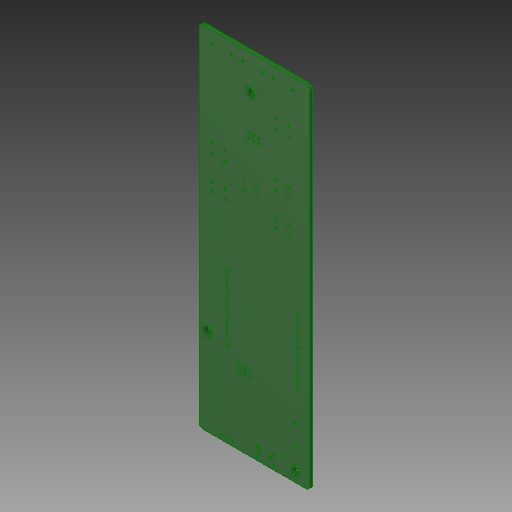
# Autodesk Inventor part: fantimote.kicad_pcb_Kontur
Saved by Autodesk Inventor 2019 (Build 230136000, 136)
## iProperties
Created: 2018-07-30
Part Number: fantimote.kicad_pcb_Kontur
Material: Generisch
Document SubType Name: Modeling
Designer: marc
Density: 1 g/cm^3
Appearance: Board-Kontur
Author: marc
Autodesk Inventor part; units mm, degrees
ref_plane "YZ Plane" through (0, 0, 0) normal (1, 0, 0) x (0, 1, 0)
ref_plane "XZ Plane" through (0, 0, 0) normal (0, 1, 0) x (-1, 0, 0)
ref_plane "XY Plane" through (0, 0, 0) normal (0, 0, 1) x (1, 0, 0)
sketch "Skizze1" plane through (0, 0, 0) normal (0, 0, 1) x (1, 0, 0)
  arc A0 (40.64, -188.595) -> (42.545, -190.5) centre (42.545, -188.595) ccw
  line L0 (42.545, -190.5) -> (93.98, -190.5)
  arc A1 (93.98, -190.5) -> (95.885, -188.595) centre (93.98, -188.595) ccw
  line L1 (95.885, -188.595) -> (95.885, -17.78)
  arc A2 (95.885, -17.78) -> (93.98, -15.875) centre (93.98, -17.78) ccw
  line L2 (93.98, -15.875) -> (42.545, -15.875)
  arc A3 (42.545, -15.875) -> (40.64, -17.78) centre (42.545, -17.78) ccw
  line L3 (40.64, -17.78) -> (40.64, -188.595)
  line L4 (70.36, -184.565) -> (70.36, -185.115)
  arc A4 (69.51, -185.115) -> (70.36, -185.115) centre (69.935, -185.115) ccw
  line L5 (69.51, -185.115) -> (69.51, -184.565)
  arc A5 (70.36, -184.565) -> (69.51, -184.565) centre (69.935, -184.565) ccw
  line L6 (77.81, -184.565) -> (77.81, -185.115)
  arc A6 (76.96, -185.115) -> (77.81, -185.115) centre (77.385, -185.115) ccw
  line L7 (76.96, -185.115) -> (76.96, -184.565)
  arc A7 (77.81, -184.565) -> (76.96, -184.565) centre (77.385, -184.565) ccw
  line L8 (70.06, -188.315) -> (70.06, -188.965)
  arc A8 (69.51, -188.965) -> (70.06, -188.965) centre (69.785, -188.965) ccw
  line L9 (69.51, -188.965) -> (69.51, -188.315)
  arc A9 (70.06, -188.315) -> (69.51, -188.315) centre (69.785, -188.315) ccw
  line L10 (77.81, -188.315) -> (77.81, -188.965)
  arc A10 (77.26, -188.965) -> (77.81, -188.965) centre (77.535, -188.965) ccw
  line L11 (77.26, -188.965) -> (77.26, -188.315)
  arc A11 (77.81, -188.315) -> (77.26, -188.315) centre (77.535, -188.315) ccw
  circle A12 centre (53.49, -85.78) radius 0.5
  circle A13 centre (46.99, -85.78) radius 0.5
  circle A14 centre (53.49, -81.28) radius 0.5
  circle A15 centre (46.99, -81.28) radius 0.5
  circle A16 centre (53.49, -69.27) radius 0.5
  circle A17 centre (46.99, -69.27) radius 0.5
  circle A18 centre (53.49, -64.77) radius 0.5
  circle A19 centre (46.99, -64.77) radius 0.5
  circle A20 centre (47.07, -21.59) radius 0.6
  circle A21 centre (57.07, -21.59) radius 0.6
  circle A22 centre (62.31, -21.59) radius 0.6
  circle A23 centre (72.31, -21.59) radius 0.6
  circle A24 centre (77.55, -21.59) radius 0.6
  circle A25 centre (87.55, -21.59) radius 0.6
  circle A26 centre (70.485, -53.34) radius 0.5
  circle A27 centre (70.485, -50.8) radius 0.5
  circle A28 centre (67.945, -53.34) radius 0.5
  circle A29 centre (67.945, -50.8) radius 0.5
  circle A30 centre (65.405, -53.34) radius 0.5
  circle A31 centre (65.405, -50.8) radius 0.5
  circle A32 centre (54.61, -115.57) radius 0.5
  circle A33 centre (54.61, -118.11) radius 0.5
  circle A34 centre (54.61, -120.65) radius 0.5
  circle A35 centre (54.61, -123.19) radius 0.5
  circle A36 centre (54.61, -125.73) radius 0.5
  circle A37 centre (54.61, -128.27) radius 0.5
  circle A38 centre (54.61, -130.81) radius 0.5
  circle A39 centre (54.61, -133.35) radius 0.5
  circle A40 centre (54.61, -135.89) radius 0.5
  circle A41 centre (54.61, -138.43) radius 0.5
  circle A42 centre (54.61, -140.97) radius 0.5
  circle A43 centre (54.61, -143.51) radius 0.5
  circle A44 centre (54.61, -146.05) radius 0.5
  circle A45 centre (54.61, -148.59) radius 0.5
  circle A46 centre (90.17, -116.205) radius 0.5
  circle A47 centre (90.17, -118.745) radius 0.5
  circle A48 centre (90.17, -121.285) radius 0.5
  circle A49 centre (90.17, -123.825) radius 0.5
  circle A50 centre (90.17, -126.365) radius 0.5
  circle A51 centre (90.17, -128.905) radius 0.5
  circle A52 centre (90.17, -131.445) radius 0.5
  circle A53 centre (90.17, -133.985) radius 0.5
  circle A54 centre (90.17, -136.525) radius 0.5
  circle A55 centre (90.17, -139.065) radius 0.5
  circle A56 centre (90.17, -141.605) radius 0.5
  circle A57 centre (90.17, -144.145) radius 0.5
  circle A58 centre (90.17, -146.685) radius 0.5
  circle A59 centre (90.17, -149.225) radius 0.5
  circle A60 centre (60.96, -153.67) radius 0.5
  circle A61 centre (60.96, -156.21) radius 0.5
  circle A62 centre (63.5, -153.67) radius 0.5
  circle A63 centre (63.5, -156.21) radius 0.5
  circle A64 centre (66.04, -153.67) radius 0.5
  circle A65 centre (66.04, -156.21) radius 0.5
  circle A66 centre (88.9, -175.1813) radius 0.5005
  circle A67 centre (88.9, -165.1787) radius 0.5005
  circle A68 centre (62.715, -72.335) radius 0.5
  circle A69 centre (69.215, -72.335) radius 0.5
  circle A70 centre (62.715, -76.835) radius 0.5
  circle A71 centre (69.215, -76.835) radius 0.5
  circle A72 centre (85.24, -42.6) radius 0.5
  circle A73 centre (78.74, -42.6) radius 0.5
  circle A74 centre (85.24, -38.1) radius 0.5
  circle A75 centre (78.74, -38.1) radius 0.5
  circle A76 centre (45.085, -146.685) radius 1.6
  circle A77 centre (47.485, -146.685) radius 0.25
  circle A78 centre (46.7821, -148.3821) radius 0.25
  circle A79 centre (45.085, -149.085) radius 0.25
  circle A80 centre (43.3879, -148.3821) radius 0.25
  circle A81 centre (42.685, -146.685) radius 0.25
  circle A82 centre (43.3879, -144.9879) radius 0.25
  circle A83 centre (45.085, -144.285) radius 0.25
  circle A84 centre (46.7821, -144.9879) radius 0.25
  circle A85 centre (88.9, -185.42) radius 1.6
  circle A86 centre (91.3, -185.42) radius 0.25
  circle A87 centre (90.5971, -187.1171) radius 0.25
  circle A88 centre (88.9, -187.82) radius 0.25
  circle A89 centre (87.2029, -187.1171) radius 0.25
  circle A90 centre (86.5, -185.42) radius 0.25
  circle A91 centre (87.2029, -183.7229) radius 0.25
  circle A92 centre (88.9, -183.02) radius 0.25
  circle A93 centre (90.5971, -183.7229) radius 0.25
  circle A94 centre (66.675, -33.02) radius 1.6
  circle A95 centre (69.075, -33.02) radius 0.25
  circle A96 centre (68.3721, -34.7171) radius 0.25
  circle A97 centre (66.675, -35.42) radius 0.25
  circle A98 centre (64.9779, -34.7171) radius 0.25
  circle A99 centre (64.275, -33.02) radius 0.25
  circle A100 centre (64.9779, -31.3229) radius 0.25
  circle A101 centre (66.675, -30.62) radius 0.25
  circle A102 centre (68.3721, -31.3229) radius 0.25
  circle A103 centre (52.07, -187.96) radius 0.45
  circle A104 centre (54.61, -187.96) radius 0.45
  circle A105 centre (57.15, -187.96) radius 0.45
  circle A106 centre (85.24, -85.78) radius 0.5
  circle A107 centre (78.74, -85.78) radius 0.5
  circle A108 centre (85.24, -81.28) radius 0.5
  circle A109 centre (78.74, -81.28) radius 0.5
  circle A110 centre (85.24, -69.27) radius 0.5
  circle A111 centre (78.74, -69.27) radius 0.5
  circle A112 centre (85.24, -64.77) radius 0.5
  circle A113 centre (78.74, -64.77) radius 0.5
  circle A114 centre (71.16, -185.89) radius 0.4
  circle A115 centre (76.16, -185.89) radius 0.4
  constraints: 116 centre point, 24 end point, 24 point on circle
extrude "fantimote.kicad_pcb_Kontur" add sketch "Skizze1" along normal blind 1.6
